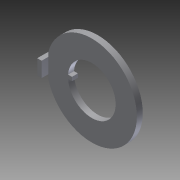
# Autodesk Inventor part: AT507H
Saved by Autodesk Inventor 2015 SP1 (Build 190203100, 203)
## iProperties
Category: PARTsolutions
Company: NKKSWITCHES
Created: 2013-12-29
Part Number: AT507H
Catalog Web Link: www.cadenas.de
Description: Locking Ring - Bushing Mount Miniature Toggles-Series M - Standard Hardwarw for Small & Large Bushings
Vendor: NKKSWITCHES
Document SubType Name: Modeling
Designer: PARTuser1
Manufacturer: NKKSWITCHES
Density: 1 g/cm^3
Material: Generic
Appearance: RGB(192.00000375509219,192.00000375509219,192.00000375509219)
PSOL_IDENT_0: {$CADENAS_DATA\23d-libs\nkkswitches\toggle\m\hardware\locking_ring.prj},194 {VTYP=3D},{NB=AT507H},{L
PSOL_IDENT_1: INA=AT507H},{NN=Locking Ring - Bushing Mount Miniature Toggles},{DATE=30.10.2007 19:43:00},{GEOMDATE
PSOL_IDENT_2: =12.04.2007 13:28:00},{VERSION=},{LINEID=10},{LINESUBID=-1},{WBVAR=}  {NB=AT507H},{LINA=AT507H},{KT=
PSOL_IDENT_3: DUMMY},{PN=AT507H},{A=0.079},{B=0.229},{D=0.472},{DD=0.250},{T=0.031},{TT=0.067},{T1=0.023},{LC=0.48
PSOL_IDENT_4: 6},{T2=0.020}
CNS_NN: Locking Ring - Bushing Mount Miniature Toggles
CNS_NT: Series M - Standard Hardwarw for Small & Large Bushings
CNS_NB: AT507H
CNS_NBSYN: $PN.
CNS_LINA: AT507H
CNS_PN: AT507H
CNS_A: 0.079
CNS_B: 0.229
CNS_D: 0.472
CNS_DD: 0.250
CNS_T: 0.031
CNS_TT: 0.067
CNS_T1: 0.023
CNS_LC: 0.486
CNS_T2: 0.020
SUPPLIER: NKKSWITCHES
ARTICLENO: AT507H
BOMINFO: AT507H
CREATOR: CADENAS GmbH
Title: AT507H
Author: Cadenas PARTsolutions
Comments: Series M - Standard Hardwarw for Small & Large Bushings
Autodesk Inventor part; units mm, degrees
sketch "Sketch_4" plane through (0, 0, 0) normal (0, 0, 1) x (1, 0, 0)
  arc A0 (-5.7658, -1.6396) -> (-5.7658, 1.6396) centre (0, 0) ccw
  line L0 (-5.7658, 1.6396) -> (-5.7658, -1.6396)
  line L1 (-3.1648, 0.254) -> (-2.6416, 0.254)
  line L2 (-2.6416, 0.254) -> (-2.6416, -0.254)
  line L3 (-2.6416, -0.254) -> (-3.1648, -0.254)
  arc A1 (-3.1648, -0.254) -> (-3.1648, 0.254) centre (0, 0) ccw
  constraints: 8 end point, 4 point on circle, 2 centre point
extrude "Extrusion1" add sketch "Sketch_4" along normal blind 0.7874
sketch "Sketch_2" plane through (0, 0, 0) normal (0, 1, 0) x (-1, 0, 0)
  line L0 (6.35, 1.7018) -> (5.7658, 1.7018)
  line L1 (5.7658, 1.7018) -> (5.7658, 0.7874)
  line L2 (5.7658, 0.7874) -> (4.4069, 0.7874)
  line L3 (4.4069, 0.7874) -> (4.4069, 0)
  line L4 (4.4069, 0) -> (5.9563, 0)
  arc A0 (5.9563, 0) -> (6.35, 0.3937) centre (5.9563, 0.3937) ccw
  line L5 (6.35, 0.3937) -> (6.35, 1.7018)
  constraints: 12 end point, 2 point on circle, 1 centre point
extrude "Extrusion2" add sketch "Sketch_2" along normal mid plane 2.0066
ref_plane "ring_XY" through (0, 0, 0.3937) normal (0, 0, 1) x (1, 0, 0)
ref_plane "ring_YZ" through (0, 0, 0.3937) normal (1, 0, 0) x (0, 1, 0)
ref_plane "ring_ZX" through (0, 0, 0.3937) normal (0, 1, 0) x (0, 0, 1)
body "Solid1"
